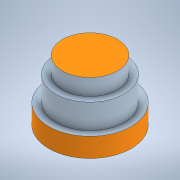
# Autodesk Inventor part: Rotor_shaft
Saved by Autodesk Inventor 2021 (Build 250183000, 183)
## iProperties
Created: 2022-07-13
Part Number: Rotor_shaft
Material: Tworzywo sztuczne PET
Document SubType Name: Modeling
Designer: MicnedSQ
Density: 1.541 g/cm^3
Appearance: Stalowoniebieska
Author: MicnedSQ
## iProperties of the stored document _Drukowanie 3D.ipt
Created: 2022-07-13
Part Number: _Drukowanie 3D
Material: Ogólny
Document SubType Name: Modeling
Designer: MicnedSQ
Density: 1 g/cm^3
Appearance: Domyślna
Author: MicnedSQ
Autodesk Inventor part; units mm, degrees
ref_plane "YZ Plane" through (0, 0, 0) normal (1, 0, 0) x (0, 1, 0)
ref_plane "XZ Plane" through (0, 0, 0) normal (0, 1, 0) x (-1, 0, 0)
ref_plane "XY Plane" through (0, 0, 0) normal (0, 0, 1) x (1, 0, 0)
sketch "Szkic1" plane through (0, 0, 0) normal (0, 1, 0) x (-1, 0, 0)
  circle A0 centre (0, 0) radius 15
  arc A1 (3.6, 1.575) -> (3.6, -1.575) centre (1.5, 0) ccw
  line L0 (3.6, -1.575) -> (3.6, 1.575)
  dimension "d0" = 30
  dimension "d1" = 5.25
  dimension "d2" = 3.6
  constraints: 2 centre point, 2 end point, 2 point on circle, 1 coincident
  measures "d0" diameter of A0
  measures "d1" diameter of A1
  measures "d2" distance from line of L0 point (0, 0)
extrude "Wyciągnięcie proste1" add sketch "Szkic1" along normal blind 20
sketch "Szkic2" plane through (0, 20, 0) normal (0, 1, 0) x (1, 0, 0)
  circle A0 centre (0, 0) radius 15 projected
  circle A1 centre (0, 0) radius 12.5
  constraints: 1 centre point, 1 coincident
extrude "Wyciągnięcie proste2" add sketch "Szkic2" against normal blind 2 contours A0 | A1
sketch "Szkic3" plane through (0, 20, 0) normal (0, 1, 0) x (1, 0, 0)
  circle A0 centre (0, 0) radius 15
  circle A1 centre (0, 0) radius 12.5
  dimension "d7" = 25
  constraints: 2 centre point, 2 coincident
  measures "d7" diameter of A1
extrude "Wyciągnięcie proste3" cut sketch "Szkic3" against normal blind 15
sketch "Szkic4" plane through (0, 20, 0) normal (0, 1, 0) x (1, 0, 0)
  circle A0 centre (0, 0) radius 10
  circle A1 centre (0, 0) radius 12.5
  dimension "d10" = 20
  constraints: 2 centre point, 2 coincident
  measures "d10" diameter of A0
extrude "Wyciągnięcie proste4" cut sketch "Szkic4" against normal blind 6
sketch "Szkic5" plane through (0, 18, 0) normal (0, -1, 0) x (1, 0, 0)
  point P0 (0, 0)
sketch "Szkic6" plane through (0, 0, 0) normal (0, -1, 0) x (1, 0, 0)
  circle A0 centre (0, 0) radius 15
  line L0 (-3.6, 1.575) -> (-3.6, -1.575) projected
  line L1 (-3.6, 1.575) -> (-3.6, -1.575)
  arc A1 (-3.6, -1.575) -> (-3.6, 1.575) centre (-1.5, 0) ccw
  constraints: 2 centre point, 2 end point, 2 point on circle, 1 coincident, 1 collinear
extrude "Wyciągnięcie proste5" add sketch "Szkic6" along normal blind 2
